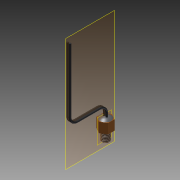
# Autodesk Inventor part: Thermistor
Saved by Autodesk Inventor 2015 (Build 190159000, 159)
## iProperties
Created: 2013-11-23
Part Number: Thermistor
Document SubType Name: Modeling
Designer: Oscar
Density: 1 g/cm^3
Material: Generic
Appearance: Bronze - Satin
Author: Oscar
Autodesk Inventor part; units mm, degrees
ref_plane "XZ Plane" through (0, 0, 0) normal (0, 1, 0) x (-1, 0, 0)
ref_plane "XY Plane" through (0, 0, 0) normal (0, 0, 1) x (1, 0, 0)
sketch "Boceto1" plane through (0, 0, 0) normal (0, 0, 1) x (1, 0, 0)
  line L0 (0, -2.702) -> (-2.34, -1.351)
  line L1 (-2.34, -1.351) -> (-2.34, 1.351)
  line L2 (-2.34, 1.351) -> (0, 2.702)
  line L3 (0, 2.702) -> (2.34, 1.351)
  line L4 (2.34, 1.351) -> (2.34, -1.351)
  line L5 (2.34, -1.351) -> (0, -2.702)
  circle A0 centre (0, 0) radius 1.5
  circle A1 centre (0, 0) radius 1.25
  dimension "d0" = 4.68
  dimension "d3" = 3
  dimension "d9" = 2.5
  constraints: 12 end point, 3 coincident, 2 centre point, 13 other
  measures "d0" distance between parallel lines of L4 L1
  measures "d3" diameter of A0
  measures "d9" diameter of A1
extrude "Extrusión1" add sketch "Boceto1" along normal blind 4 contours L0 L1 L2 L3 L4 L5 | A0 | A1
extrude "Extrusión2" add sketch "Boceto1" against normal blind 4 contours A0 | A1
chamfer "Chaflán1" distance 0.25 angle 45 1 edges at (-1.5, 0, -4)
extrude "Extrusión3" cut sketch "Boceto1" against normal blind 0.5 contours A0
thread "Rosca1"
sketch "Boceto2" plane through (0, 0, 0) normal (1, 0, 0) x (0, 1, 0)
  line L0 (1.351, 4) -> (-1.351, 4) projected
  line L1 (0, 4) -> (2.25, 4)
  line L2 (0, 4) -> (0, 4.75)
  arc A0 (2.25, 4) -> (0, 4.75) centre (0, 1) ccw
  dimension "d14" = 0.75
  dimension "d15" = 4.5
  constraints: 4 end point, 2 point on circle, 2 point on line, 1 centre point, 1 midpoint, 1 perpendicular
  measures "d14" distance of L1.start L2.end
  measures "d15" diameter of L1.end L2
revolve "Revolución1" add sketch "Boceto2" angle 360 about axis through (0, 0, 4) along (0, 0, 1)
ref_plane "Plano de trabajo1" through (-0.5, 0, 0) normal (1, 0, 0) x (0, 1, 0)
sketch "Boceto4" plane through (0, 0, 4) normal (0, 0, 1) x (1, 0, 0)
  circle A0 centre (-0.5, 0) radius 0.375
  dimension "d21" = 0.75
  constraints: 1 centre point, 1 coincident
  measures "d21" diameter of A0
sketch "Boceto3" plane through (-0.5, 0, 0) normal (1, 0, 0) x (0, 1, 0)
  line L0 (1.351, 4) -> (-1.351, 4) projected
  line L1 (0, 4) -> (0, 6)
  arc A0 (0, 6) -> (-3, 9) centre (-3, 6) ccw
  line L2 (-3, 9) -> (-12, 9)
  arc A1 (-15, 12) -> (-12, 9) centre (-12, 12) ccw
  line L3 (-15, 12) -> (-15, 38.107)
  dimension "d18" = 2
  dimension "d19" = 5
  dimension "d20" = 15
  constraints: 6 end point, 4 point on circle, 4 tangent, 2 centre point, 2 perpendicular, 1 equal radius, 1 midpoint, 1 parallel
  measures "d18" distance of L1.start L1.end
  measures "d19" distance between parallel lines of L0 L2
  measures "d20" distance between parallel lines of L3 L1
sweep "Barrido1" add profiles "Boceto4" path "Boceto3" path curves L1 A0 L2 A1 L3
mirror "Simetría1" about plane through (0, 0, 0) normal (1, 0, 0) of "Barrido1"
body "Solid1"
